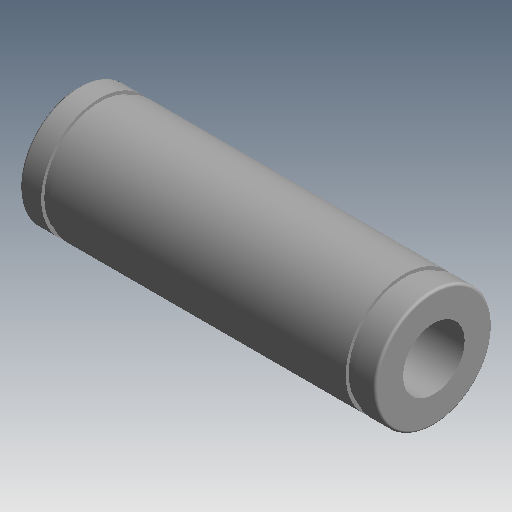
# Autodesk Inventor part: BUSHING_REFERENCE_DATA_FOR_LHSSW10
Saved by Autodesk Inventor 2020 (Build 240168000, 168)
## iProperties
Part Number: BUSHING_REFERENCE_DATA_FOR_LHSSW10
Material: 一般
Catalog Web Link: www.cadenas.de
Description: BUSHING_REFERENCE_DATA_FOR_LHSSW-Linear Bushings - Double Type For LHSSW
Vendor: MISUMI
Document SubType Name: Modeling
Designer: partserver
Manufacturer: MISUMI
Mass: 11.7482 g
Surface Area: 57.5424 cm^2
Volume: 11.7482 cm^3
Density: 1 g/cm^3
Appearance: PSOLRGB-192-192-192
Category: PARTsolutions
Company: MISUMI
PSOL_IDENT_0: {$CADENAS_DATA\23d-libs\misumi\metric\04_linear_bushings\lhssw\lhssw_lmu.prj},235 {VTYP=3D},{NB=BUSH
PSOL_IDENT_1: ING_REFERENCE_DATA_FOR_LHSSW10},{LINA=BUSHING_REFERENCE_DATA_FOR_LHSSW10},{NN=BUSHING_REFERENCE_DATA
PSOL_IDENT_2: _FOR_LHSSW},{DATE=30.11.2021 05:42:29},{GEOMDATE=13.03.2015 00:48:00},{VERSION=},{LINEID=100},{WBVAR=
PSOL_IDENT_3: },{WBNUMERIC=}  {NB=BUSHING_REFERENCE_DATA_FOR_LHSSW10},{LINA=BUSHING_REFERENCE_DATA_FOR_LHSSW10},{K
PSOL_IDENT_4: T=DUMMY},{PN=BUSHING_REFERENCE_DATA_FOR_LHSSW10},{TYPE=BUSHING_REFERENCE_DATA_FOR_LHSSW},{DDRR=10},{
PSOL_IDENT_5: D=19},{LLB=29},{LH=68},{SH=4.0},{RRW=1.15},{B=19.4},{W=1.30},{D1=18.0},{RR=0.4}
NB: BUSHING_REFERENCE_DATA_FOR_LHSSW10
NN: BUSHING_REFERENCE_DATA_FOR_LHSSW
NT: Linear Bushings - Double Type For LHSSW
NBSYN: $PN.
LINA: BUSHING_REFERENCE_DATA_FOR_LHSSW10
CATALOG: Misumi
PN: BUSHING_REFERENCE_DATA_FOR_LHSSW10
DDRR: 10
D: 19
LLB: 29
LH: 68
SH: 4
RRW: 1.15
B: 19.4
W: 1.3
D1: 18
RR: 0.4
SUPPLIER: MISUMI
ARTICLENO: BUSHING_REFERENCE_DATA_FOR_LHSSW10
BOMINFO: BUSHING_REFERENCE_DATA_FOR_LHSSW10
CREATOR: CADENAS GmbH
Title: BUSHING_REFERENCE_DATA_FOR_LHSSW10
Author: Cadenas PARTsolutions
Comments: Linear Bushings - Double Type For LHSSW
Autodesk Inventor part; units mm, degrees
sketch "Sketch_1" plane through (0, 0, 0) normal (0, 0, 1) x (1, 0, 0)
  line L0 (28.85, 0) -> (-28.85, 0)
  line L1 (-28.85, 0) -> (-28.85, 9.1)
  arc A0 (-28.45, 9.5) -> (-28.85, 9.1) centre (-28.45, 9.1) ccw
  line L2 (-28.45, 9.5) -> (-25.35, 9.5)
  line L3 (-25.35, 9.5) -> (-25.35, 9)
  line L4 (-25.35, 9) -> (-24.05, 9)
  line L5 (-24.05, 9) -> (-24.05, 9.5)
  line L6 (-24.05, 9.5) -> (24.05, 9.5)
  line L7 (24.05, 9.5) -> (24.05, 9)
  line L8 (24.05, 9) -> (25.35, 9)
  line L9 (25.35, 9) -> (25.35, 9.5)
  line L10 (25.35, 9.5) -> (28.45, 9.5)
  arc A1 (28.85, 9.1) -> (28.45, 9.5) centre (28.45, 9.1) ccw
  line L11 (28.85, 9.1) -> (28.85, 0)
  line L12 (28.85, 0) -> (-28.85, 0)
  constraints: 26 end point, 4 point on circle, 2 centre point
revolve "Revolution1" add sketch "Sketch_1" angle 360 about axis through (28.85, 0, 0) along (1, 0, 0)
sketch "Sketch2" plane through (28.85, 0, 0) normal (1, 0, 0) x (0, 0, -1)
  point P0 (0, 0)
hole "Hole1" at (28.85, 0, 0) direction (-1, 0, 0) diameter 10 depth 57.7
ref_plane "to_housing_XY" through (0, 0, 0) normal (-1, 0, 0) x (0, 0, -1)
ref_plane "to_housing_YZ" through (0, 0, 0) normal (0, 0, -1) x (0, -1, 0)
ref_plane "to_housing_ZX" through (0, 0, 0) normal (0, -1, 0) x (-1, 0, 0)
body "Solid1"
